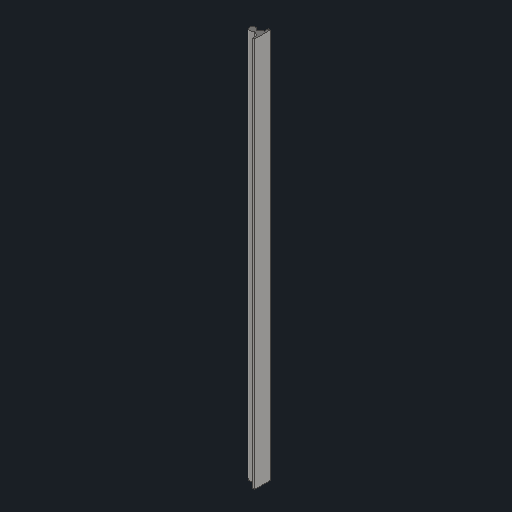
# Autodesk Inventor part: rail
Saved by Autodesk Inventor 2026.3 (Build 303398000, 398)
## iProperties
Created: 2026-06-05
Part Number: rail
Material: ステンレス鋼 440C
Document SubType Name: Modeling
Designer: shusu
Density: 7.75 g/cm^3
Appearance: 半つや出し
Author: shusu
Autodesk Inventor part; units mm, degrees
ref_plane "YZ Plane" through (0, 0, 0) normal (1, 0, 0) x (0, 1, 0)
ref_plane "XZ Plane" through (0, 0, 0) normal (0, 1, 0) x (-1, 0, 0)
ref_plane "XY Plane" through (0, 0, 0) normal (0, 0, 1) x (1, 0, 0)
sketch "スケッチ1" plane through (0, 0, 0) normal (0, 1, 0) x (-1, 0, 0)
  circle A0 centre (0, 0) radius 8
  line L0 (0, 0) -> (-25, 0)
  line L1 (-25, 0) -> (-25, 20)
  line L2 (-25, 20) -> (-20, 20)
  line L3 (-20, 20) -> (-20, 10)
  line L4 (-20, 10) -> (-7.5002, 2.7833)
  line L5 (-25, 0) -> (-25, -20)
  line L6 (-25, -20) -> (-20, -20)
  line L7 (-20, -20) -> (-20, -10)
  line L8 (-20, -10) -> (-7.5002, -2.7833)
  dimension "d0" = 16
  dimension "d1" = 25
  dimension "d2" = 20
  dimension "d3" = 5
  constraints: 18 end point, 4 symmetric about line, 2 perpendicular, 1 coincident, 1 horizontal, 1 vertical, 3 other
  measures "d1" distance of L0.start L0.end
  measures "d2" distance of L0.end L1.end
  measures "d3" distance of L1.end L2.end
extrude "押し出し1" add sketch "スケッチ1" along normal blind 1000
